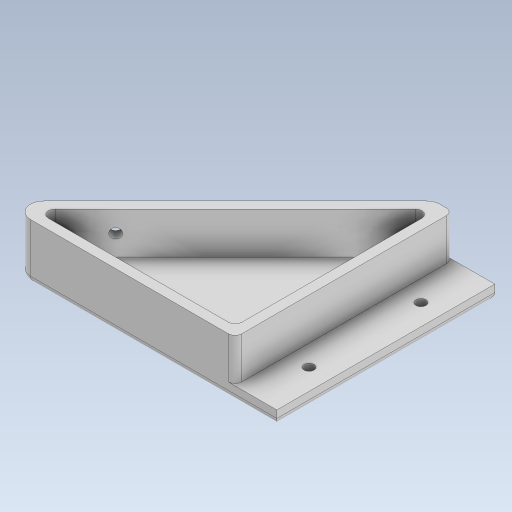
# Autodesk Inventor part: Part1
Saved by Autodesk Inventor 2023 (Build 270158000, 158)
## iProperties
Created: 2023-04-04
Part Number: Part1
Material: Generic
Document SubType Name: Modeling
Designer: Dave
Density: 1 g/cm^3
Appearance: Default
Author: Dave
## iProperties of the stored document Part1_3DPrint.ipt
Created: 2023-04-04
Part Number: Part1_3DPrint
Material: Generic
Document SubType Name: Modeling
Designer: Dave
Density: 1 g/cm^3
Appearance: Default
Author: Dave
Autodesk Inventor part; units mm, degrees
ref_plane "YZ Plane" through (0, 0, 0) normal (1, 0, 0) x (0, 1, 0)
ref_plane "XZ Plane" through (0, 0, 0) normal (0, 1, 0) x (-1, 0, 0)
ref_plane "XY Plane" through (0, 0, 0) normal (0, 0, 1) x (1, 0, 0)
sketch "Sketch1" plane through (0, 0, 0) normal (0, 1, 0) x (-1, 0, 0)
  line L0 (0, -6.35) -> (0, -98.0626)
  line L1 (10.8401, -102.5527) -> (102.5527, -10.8401)
  line L2 (98.0626, 0) -> (6.35, 0)
  arc A0 (102.5527, -10.8401) -> (98.0626, 0) centre (98.0626, -6.35) ccw
  arc A1 (0, -98.0626) -> (10.8401, -102.5527) centre (6.35, -98.0626) ccw
  arc A2 (6.35, 0) -> (0, -6.35) centre (6.35, -6.35) ccw
  line L3 (0, 0) -> (-20, 0)
  line L4 (-20, 0) -> (-20, -104.4126)
  line L5 (-20, -104.4126) -> (0, -104.4126)
  line L6 (0, -104.4126) -> (0, 0)
  line L7 (0, 0) -> (6.35, 0)
  line L8 (0, -104.4126) -> (6.35, -104.4126)
  point P0 (113.3929, 0)
  dimension "d0" = 113.3929
  dimension "d1" = 6.35
  dimension "d8" = 20
  constraints: 18 end point, 9 tangent, 7 point on circle, 4 point on line, 3 centre point, 3 perpendicular, 2 equal radius, 2 horizontal, 2 parallel, 1 vertical
  measures "d0" distance of point (113.393, 0) L3.start
  measures "d1" radius of A0
  measures "d8" distance of L4.end L5.end
extrude "Extrusion1" add sketch "Sketch1" along normal blind 6.6929
sketch "Sketch2" plane through (0, 6.6929, 0) normal (0, 1, 0) x (1, 0, 0)
  arc A0 (-6.35, 104.4126) -> (-10.8401, 102.5527) centre (-6.35, 98.0626) ccw projected
  line L0 (-10.8401, 102.5527) -> (-102.5527, 10.8401) projected
  arc A1 (-102.5527, 10.8401) -> (-98.0626, 0) centre (-98.0626, 6.35) ccw projected
  line L1 (-4.7625, 4.7625) -> (-104.211, 4.7625)
  line L2 (-101.8952, 4.7625) -> (-4.7625, 101.8952)
  line L3 (-4.7625, 104.211) -> (-4.7625, 4.7625)
  line L4 (-98.0626, 0) -> (20, 0) projected
  line L5 (20, 0) -> (20, 104.4126) projected
  line L6 (20, 104.4126) -> (-6.35, 104.4126) projected
  line L7 (0, 0) -> (0, 104.4126)
  point P0 (0, 0)
  constraints: 8 end point, 3 point on line, 2 point on circle, 1 perpendicular
extrude "Extrusion2" add sketch "Sketch2" along normal blind 20 contours L6 L7 L4 A1 L0 A0
sketch "Sketch3" plane through (0, 6.6929, 0) normal (0, 1, 0) x (1, 0, 0)
  circle A0 centre (10, 25.4) radius 2.4193
  circle A1 centre (10, 79.0126) radius 2.4193
  line L0 (20, 0) -> (20, 104.4126) projected
  line L1 (0, 0) -> (20, 0) projected
  dimension "d9" = 10
  dimension "d10" = 25.4
  dimension "d11" = 25.4
  dimension "d12" = 4.8387
  constraints: 2 centre point, 1 equal radius, 1 vertical alignment
  measures "d9" distance from line of L0 A0.centre
  measures "d10" distance from line of L1 A0.centre
  measures "d11" vertical distance of A1.centre L0.end
  measures "d12" diameter of A0
extrude "Extrusion3" cut sketch "Sketch3" against normal blind 12.954
sketch "Sketch5" plane through (-102.5527, 0, -10.8401) normal (-0.7071068, 0, -0.7071068) x (-0.7071068, 0, 0.7071068)
  circle A0 centre (-24.3815, 16.6929) radius 2.3813
  line L0 (-138.6815, 6.6929) -> (-138.6815, 26.6929) projected
  line L1 (-129.7012, 26.6929) -> (0, 26.6929) projected
  line L2 (-129.7012, 0) -> (0, 0) projected
  line L3 (-152.8236, 6.6929) -> (-138.6815, 6.6929) projected
  line L4 (-78.9927, 0) -> (-152.8236, 0) projected
  point P0 (-64.8506, 0)
  dimension "d15" = 114.3
  dimension "d17" = 16.6929
  dimension "d18" = 6.6929
  dimension "d19" = 4.7625
  constraints: 1 centre point
  measures "d15" distance from line of L0 A0.centre
  measures "d17" distance from line of A0.centre L2
  measures "d18" distance between parallel lines of L3 L4
  measures "d19" diameter of A0
extrude "Extrusion4" cut sketch "Sketch5" against normal up to surface (4.7625 mm away)
fillet "Fillet1" radius 3.175 11 edges at (-4.7625, 16.6929, -4.7625) (-101.8952, 16.6929, -4.7625) (-4.7625, 16.6929, -101.8952) (0, 16.6929, -104.4126) (-8.78, 0, -103.9292) (-56.6964, 0, -56.6964) (-103.9292, 0, -3.92) (-39.0313, 0, 0) (6.825, 0, -104.4126) (20, 0, -52.2063) (0, 16.6929, 0)
body "Solid1"
